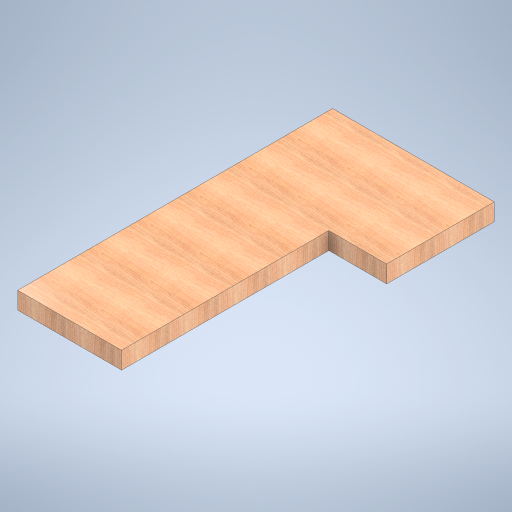
# Autodesk Inventor part: Stand--Sink_and_Corner_Cabinets
Saved by Autodesk Inventor 2024 (Build 280153000, 153)
## iProperties
Created: 2023-03-29
Part Number: Stand--Sink_and_Corner_Cabinets
Material: Wood (Birch)
Document SubType Name: Modeling
Designer: Tom
Density: 0.55 g/cm^3
Appearance: Birch - Natural Polished
Author: Tom
Autodesk Inventor part; units mm, degrees
ref_plane "YZ Plane" through (0, 0, 0) normal (1, 0, 0) x (0, 1, 0)
ref_plane "XZ Plane" through (0, 0, 0) normal (0, 1, 0) x (-1, 0, 0)
ref_plane "XY Plane" through (0, 0, 0) normal (0, 0, 1) x (1, 0, 0)
sketch "Sketch1" plane through (0, 0, 0) normal (0, 1, 0) x (-1, 0, 0)
  line L0 (536.575, 1069.975) -> (0, 1069.975)
  line L1 (0, 1069.975) -> (0, 0)
  line L2 (0, 0) -> (-298.45, 0)
  line L3 (-298.45, 0) -> (-298.45, -555.625)
  line L4 (-298.45, -555.625) -> (536.575, -555.625)
  line L5 (536.575, -555.625) -> (536.575, 1069.975)
  dimension "d1" = 536.575
  dimension "d2" = 835.025
  dimension "d3" = 555.625
  dimension "d9" = 1069.975
  dimension "d10" = 1625.6
  dimension "d11" = 298.45
  constraints: 12 end point, 2 parallel, 1 coincident, 1 horizontal, 1 perpendicular
  measures "d1" distance of L0.start L0.end
  measures "d2" distance of L3.end L4.end
  measures "d3" distance of L2.end L3.end
  measures "d9" distance of L0.end L1.end
  measures "d10" distance of L4.end L0.start
  measures "d11" distance of L1.end L2.end
extrude "Extrusion1" add sketch "Sketch1" along normal blind 88.9
body "Solid1"
